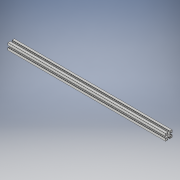
# Autodesk Inventor part: 500mm 2020
Saved by Autodesk Inventor 2018 (Build 220112000, 112)
## iProperties
Created: 2019-01-19
Part Number: 500mm 2020
Material: Generic
Document SubType Name: Sheet Metal
Designer: User
Density: 1 g/cm^3
Sheet Metal Rule: 기본값
Appearance: Default
Author: User
Autodesk Inventor part; units mm, degrees
ref_plane "YZ Plane" through (0, 0, 0) normal (1, 0, 0) x (0, 1, 0)
ref_plane "XZ Plane" through (0, 0, 0) normal (0, 1, 0) x (-1, 0, 0)
ref_plane "XY Plane" through (0, 0, 0) normal (0, 0, 1) x (1, 0, 0)
sketch "Sketch1" plane through (0, 0, 0) normal (1, 0, 0) x (0, 1, 0)
  line L0 (9.5486, -7.0751) -> (4.5486, -7.0751)
  line L1 (7.0486, -9.5751) -> (7.0486, -4.5751)
  circle A0 centre (7.0486, -7.0751) radius 2
  circle A1 centre (7.0486, 6.9249) radius 2
  line L2 (7.0486, 9.4249) -> (7.0486, 4.4249)
  line L3 (9.5486, 6.9249) -> (4.5486, 6.9249)
  line L4 (4.1986, 4.8676) -> (4.1986, 8.1249)
  arc A2 (4.1986, 8.1249) -> (3.8986, 8.4249) centre (3.8986, 8.1249) ccw
  line L5 (3.8986, 8.4249) -> (2.9986, 8.4249)
  arc A3 (2.6986, 8.7249) -> (2.9986, 8.4249) centre (2.9986, 8.7249) ccw
  line L6 (2.6986, 8.7249) -> (2.6986, 9.6249)
  arc A4 (2.9986, 9.9249) -> (2.6986, 9.6249) centre (2.9986, 9.6249) ccw
  line L7 (2.9986, 9.9249) -> (9.7486, 9.9249)
  arc A5 (10.0486, 9.6249) -> (9.7486, 9.9249) centre (9.7486, 9.6249) ccw
  line L8 (10.0486, 9.6249) -> (10.0486, 2.8749)
  arc A6 (9.7486, 2.5749) -> (10.0486, 2.8749) centre (9.7486, 2.8749) ccw
  line L9 (9.7486, 2.5749) -> (8.8486, 2.5749)
  arc A7 (8.5486, 2.8749) -> (8.8486, 2.5749) centre (8.8486, 2.8749) ccw
  line L10 (8.5486, 2.8749) -> (8.5486, 3.7749)
  arc A8 (8.5486, 3.7749) -> (8.2486, 4.0749) centre (8.2486, 3.7749) ccw
  line L11 (8.2486, 4.0749) -> (4.9914, 4.0749)
  arc A9 (4.9914, 4.0749) -> (4.7564, 3.9614) centre (4.9914, 3.7749) ccw
  arc A10 (4.7564, 3.9614) -> (3.3559, 0.2322) centre (9.8395, -0.0751) ccw
  line L12 (3.3559, 0.2322) -> (3.0486, -0.0751)
  line L13 (3.0486, -0.0751) -> (3.3559, -0.3824)
  arc A11 (3.3559, -0.3824) -> (4.7564, -4.1117) centre (9.8395, -0.0751) ccw
  arc A12 (4.7564, -4.1117) -> (4.9914, -4.2251) centre (4.9914, -3.9251) ccw
  line L14 (4.9914, -4.2251) -> (8.2486, -4.2251)
  arc A13 (8.2486, -4.2251) -> (8.5486, -3.9251) centre (8.2486, -3.9251) ccw
  line L15 (8.5486, -3.9251) -> (8.5486, -3.0251)
  arc A14 (8.8486, -2.7251) -> (8.5486, -3.0251) centre (8.8486, -3.0251) ccw
  line L16 (8.8486, -2.7251) -> (9.7486, -2.7251)
  arc A15 (10.0486, -3.0251) -> (9.7486, -2.7251) centre (9.7486, -3.0251) ccw
  line L17 (10.0486, -3.0251) -> (10.0486, -9.7751)
  arc A16 (9.7486, -10.0751) -> (10.0486, -9.7751) centre (9.7486, -9.7751) ccw
  line L18 (9.7486, -10.0751) -> (2.9986, -10.0751)
  arc A17 (2.6986, -9.7751) -> (2.9986, -10.0751) centre (2.9986, -9.7751) ccw
  line L19 (2.6986, -9.7751) -> (2.6986, -8.8751)
  arc A18 (2.9986, -8.5751) -> (2.6986, -8.8751) centre (2.9986, -8.8751) ccw
  line L20 (2.9986, -8.5751) -> (3.8986, -8.5751)
  arc A19 (3.8986, -8.5751) -> (4.1986, -8.2751) centre (3.8986, -8.2751) ccw
  line L21 (4.1986, -8.2751) -> (4.1986, -5.0179)
  arc A20 (4.1986, -5.0179) -> (4.0852, -4.7829) centre (3.8986, -5.0179) ccw
  arc A21 (4.0852, -4.7829) -> (0.3559, -3.3824) centre (0.0486, -9.8659) ccw
  line L22 (0.3559, -3.3824) -> (0.0486, -3.0751)
  line L23 (0.0486, -3.0751) -> (-0.2587, -3.3824)
  arc A22 (-0.2587, -3.3824) -> (-3.9879, -4.7829) centre (0.0486, -9.8659) ccw
  arc A23 (-3.9879, -4.7829) -> (-4.1014, -5.0179) centre (-3.8014, -5.0179) ccw
  line L24 (-4.1014, -5.0179) -> (-4.1014, -8.2751)
  arc A24 (-4.1014, -8.2751) -> (-3.8014, -8.5751) centre (-3.8014, -8.2751) ccw
  line L25 (-3.8014, -8.5751) -> (-2.9014, -8.5751)
  arc A25 (-2.6014, -8.8751) -> (-2.9014, -8.5751) centre (-2.9014, -8.8751) ccw
  line L26 (-2.6014, -8.8751) -> (-2.6014, -9.7751)
  arc A26 (-2.9014, -10.0751) -> (-2.6014, -9.7751) centre (-2.9014, -9.7751) ccw
  line L27 (-2.9014, -10.0751) -> (-9.6514, -10.0751)
  arc A27 (-9.9514, -9.7751) -> (-9.6514, -10.0751) centre (-9.6514, -9.7751) ccw
  line L28 (-9.9514, -9.7751) -> (-9.9514, -3.0251)
  arc A28 (-9.6514, -2.7251) -> (-9.9514, -3.0251) centre (-9.6514, -3.0251) ccw
  line L29 (-9.6514, -2.7251) -> (-8.7514, -2.7251)
  arc A29 (-8.4514, -3.0251) -> (-8.7514, -2.7251) centre (-8.7514, -3.0251) ccw
  line L30 (-8.4514, -3.0251) -> (-8.4514, -3.9251)
  arc A30 (-8.4514, -3.9251) -> (-8.1514, -4.2251) centre (-8.1514, -3.9251) ccw
  line L31 (-8.1514, -4.2251) -> (-4.8941, -4.2251)
  arc A31 (-4.8941, -4.2251) -> (-4.6592, -4.1117) centre (-4.8941, -3.9251) ccw
  arc A32 (-4.6592, -4.1117) -> (-3.2587, -0.3824) centre (-9.7422, -0.0751) ccw
  line L32 (-3.2587, -0.3824) -> (-2.9514, -0.0751)
  line L33 (-2.9514, -0.0751) -> (-3.2587, 0.2322)
  arc A33 (-3.2587, 0.2322) -> (-4.6592, 3.9614) centre (-9.7422, -0.0751) ccw
  arc A34 (-4.6592, 3.9614) -> (-4.8941, 4.0749) centre (-4.8941, 3.7749) ccw
  line L34 (-4.8941, 4.0749) -> (-8.1514, 4.0749)
  arc A35 (-8.1514, 4.0749) -> (-8.4514, 3.7749) centre (-8.1514, 3.7749) ccw
  line L35 (-8.4514, 3.7749) -> (-8.4514, 2.8749)
  arc A36 (-8.7514, 2.5749) -> (-8.4514, 2.8749) centre (-8.7514, 2.8749) ccw
  line L36 (-8.7514, 2.5749) -> (-9.6514, 2.5749)
  arc A37 (-9.9514, 2.8749) -> (-9.6514, 2.5749) centre (-9.6514, 2.8749) ccw
  line L37 (-9.9514, 2.8749) -> (-9.9514, 9.6249)
  arc A38 (-9.6514, 9.9249) -> (-9.9514, 9.6249) centre (-9.6514, 9.6249) ccw
  line L38 (-9.6514, 9.9249) -> (-2.9014, 9.9249)
  arc A39 (-2.6014, 9.6249) -> (-2.9014, 9.9249) centre (-2.9014, 9.6249) ccw
  line L39 (-2.6014, 9.6249) -> (-2.6014, 8.7249)
  arc A40 (-2.9014, 8.4249) -> (-2.6014, 8.7249) centre (-2.9014, 8.7249) ccw
  line L40 (-2.9014, 8.4249) -> (-3.8014, 8.4249)
  arc A41 (-3.8014, 8.4249) -> (-4.1014, 8.1249) centre (-3.8014, 8.1249) ccw
  line L41 (-4.1014, 8.1249) -> (-4.1014, 4.8676)
  arc A42 (-4.1014, 4.8676) -> (-3.9879, 4.6327) centre (-3.8014, 4.8676) ccw
  arc A43 (-3.9879, 4.6327) -> (-0.2587, 3.2322) centre (0.0486, 9.7157) ccw
  line L42 (-0.2587, 3.2322) -> (0.0486, 2.9249)
  line L43 (0.0486, 2.9249) -> (0.3559, 3.2322)
  arc A44 (0.3559, 3.2322) -> (4.0852, 4.6327) centre (0.0486, 9.7157) ccw
  arc A45 (4.0852, 4.6327) -> (4.1986, 4.8676) centre (3.8986, 4.8676) ccw
  line L44 (-11.1503, -0.0751) -> (11.2475, -0.0751)
  circle A46 centre (0.0486, -0.0751) radius 2.15
  circle A47 centre (-6.9514, -7.0751) radius 2
  line L45 (-6.9514, -9.5751) -> (-6.9514, -4.5751)
  line L46 (-9.4514, -7.0751) -> (-4.4514, -7.0751)
  circle A48 centre (-6.9514, 6.9249) radius 2
  line L47 (-6.9514, 9.4249) -> (-6.9514, 4.4249)
  line L48 (-9.4514, 6.9249) -> (-4.4514, 6.9249)
  constraints: 98 end point, 88 point on circle, 49 centre point, 2 point on line
extrude "Extrusion1" add sketch "Sketch1" along normal blind 470
equation "\"BendRadius\" = Thickness"
equation "\"BendReliefWidth\" = Thickness"
equation "\"BendReliefDepth\" = 0.5 * Thickness"
equation "\"CornerReliefSize\" = 4 * Thickness"
equation "\"MinimumRemnant\" = 2 * Thickness"
equation "\"TransitionRadius\" = BendRadius"
equation "\"JacobiRadiusSize\" = BendRadius"
equation "\"GapSize\" = Thickness"
equation "\"Thickness\" = 3.048"
body "Solid1"
